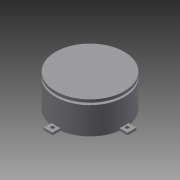
# Autodesk Inventor part: Rotating Base
Saved by Autodesk Inventor 2014 (Build 180170000, 170)
## iProperties
Created: 2015-07-31
Part Number: Rotating Base
Material: Generic
Document SubType Name: Modeling
Designer: Devon
Density: 1 g/cm^3
Appearance: Default
Author: Devon
Autodesk Inventor part; units mm, degrees
ref_plane "YZ Plane" through (0, 0, 0) normal (1, 0, 0) x (0, 1, 0)
ref_plane "XZ Plane" through (0, 0, 0) normal (0, 1, 0) x (-1, 0, 0)
ref_plane "XY Plane" through (0, 0, 0) normal (0, 0, 1) x (1, 0, 0)
sketch "Sketch1" plane through (0, 0, 0) normal (0, 1, 0) x (-1, 0, 0)
  circle A0 centre (53.5305, 0) radius 2.3813
  circle A1 centre (0, -53.5305) radius 2.3876
  circle A2 centre (-53.5305, 0) radius 2.3876
  circle A3 centre (0, 53.5305) radius 2.3876
  line L0 (0, 60.2361) -> (-6.35, 60.2361)
  line L1 (-6.35, 60.2361) -> (6.35, 60.2361)
  line L2 (6.35, 60.2361) -> (6.35, 48.8011)
  line L3 (-6.35, 60.2361) -> (-6.35, 48.8011)
  line L4 (-60.2361, 0) -> (-60.2361, -6.35)
  line L5 (-60.2361, -6.35) -> (-60.2361, 6.35)
  line L6 (-60.2361, 6.35) -> (-48.8011, 6.35)
  line L7 (-60.2361, -6.35) -> (-48.8011, -6.35)
  line L8 (0, -60.2361) -> (-6.35, -60.2361)
  line L9 (-6.35, -60.2361) -> (6.35, -60.2361)
  line L10 (6.35, -60.2361) -> (6.35, -48.8011)
  line L11 (-6.35, -60.2361) -> (-6.35, -48.8011)
  line L12 (60.2361, 0) -> (60.2361, -6.35)
  line L13 (60.2361, -6.35) -> (60.2361, 6.35)
  line L14 (60.2361, 6.35) -> (48.8011, 6.35)
  line L15 (60.2361, -6.35) -> (48.8011, -6.35)
  arc A4 (6.35, -48.8011) -> (48.8011, -6.35) centre (0, 0) ccw
  arc A5 (-48.8011, -6.35) -> (-6.35, -48.8011) centre (0, 0) ccw
  arc A6 (48.8011, 6.35) -> (6.35, 48.8011) centre (0, 0) ccw
  arc A7 (-6.35, 48.8011) -> (-48.8011, 6.35) centre (0, 0) ccw
  circle A8 centre (0, 0) radius 49.2125
  dimension "d6" = 4.7625
  dimension "d7" = 4.7752
  dimension "d8" = 4.7752
  dimension "d9" = 4.7752
  dimension "d11" = 6.7056
  dimension "d12" = 6.7056
  dimension "d13" = 6.7056
  dimension "d14" = 6.7056
  dimension "d15" = 6.35
  dimension "d16" = 12.7
  dimension "d17" = 6.35
  dimension "d18" = 12.7
  dimension "d19" = 6.35
  dimension "d20" = 12.7
  dimension "d21" = 6.35
  dimension "d22" = 12.7
  constraints: 32 end point, 9 centre point, 8 point on circle, 6 parallel, 3 collinear, 3 perpendicular, 2 coincident, 1 concentric
  measures "d6" diameter of A0
  measures "d7" diameter of A1
  measures "d8" diameter of A2
  measures "d9" diameter of A3
  measures "d11" distance of A2.centre L4.start
  measures "d12" distance of A1.centre L8.start
  measures "d13" distance of A0.centre L12.start
  measures "d14" distance of A3.centre L0.start
  measures "d15" distance of L0.start L0.end
  measures "d16" distance of L0.end L1.end
  measures "d17" distance of L4.start L4.end
  measures "d18" distance of L4.end L5.end
  measures "d19" distance of L8.start L8.end
  measures "d20" distance of L8.end L9.end
  measures "d21" distance of L12.start L12.end
  measures "d22" distance of L12.end L13.end
extrude "Extrusion1" add sketch "Sketch1" along normal blind 3.175
sketch "Sketch2" plane through (0, 3.175, 0) normal (0, 1, 0) x (1, 0, 0)
  arc A0 (48.8011, 6.35) -> (6.35, 48.8011) centre (0, 0) ccw projected
  arc A1 (-48.8011, -6.35) -> (-6.35, -48.8011) centre (0, 0) ccw projected
  circle A2 centre (0, 0) radius 49.2125
  constraints: 1 centre point, 1 coincident, 1 concentric
extrude "Extrusion2" add sketch "Sketch2" along normal blind 35.7188
sketch "Sketch3" plane through (0, 38.8937, 0) normal (0, 1, 0) x (1, 0, 0)
  circle A0 centre (0, 0) radius 49.2125 projected
  circle A1 centre (0, 0) radius 6.35
  dimension "d27" = 12.7
  constraints: 1 centre point, 1 coincident
  measures "d27" diameter of A1
extrude "Extrusion3" add sketch "Sketch3" along normal blind 3.175 contours A1
sketch "Sketch4" plane through (0, 42.0688, 0) normal (0, 1, 0) x (1, 0, 0)
  circle A0 centre (0, 0) radius 6.35 projected
  circle A1 centre (0, 0) radius 49.2125
  dimension "d30" = 98.425
  constraints: 1 centre point, 1 coincident
  measures "d30" diameter of A1
extrude "Extrusion4" add sketch "Sketch4" along normal blind 3.9688 contours A0 | A1
body "Solid1"
